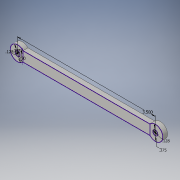
# Autodesk Inventor part: Sun_LinkageArm
Saved by Autodesk Inventor 2016 (Build 200138000, 138)
## iProperties
Created: 2018-01-10
Part Number: Sun_LinkageArm
Material: Generic
Document SubType Name: Modeling
Designer: sun01147
Density: 1 g/cm^3
Appearance: Default
Mass: 2.01542 g
Surface Area: 19.9973 cm^2
Volume: 2.01542 cm^3
Author: sun01147
Autodesk Inventor part; units mm, degrees
ref_plane "YZ Plane" through (0, 0, 0) normal (1, 0, 0) x (0, 1, 0)
ref_plane "XZ Plane" through (0, 0, 0) normal (0, 1, 0) x (-1, 0, 0)
ref_plane "XY Plane" through (0, 0, 0) normal (0, 0, 1) x (1, 0, 0)
sketch "Linkagearm" plane through (0, 0, 0) normal (0, 0, 1) x (1, 0, 0)
  arc A0 (3.5498, 3.175) -> (3.5498, -3.175) centre (0, 0) ccw
  line L0 (3.5498, 3.175) -> (85.3502, 3.175)
  line L1 (85.3502, 3.175) -> (85.3502, -3.175)
  line L2 (85.3502, -3.175) -> (3.5498, -3.175)
  line L3 (3.5498, -3.175) -> (3.5498, 3.175)
  arc A1 (85.3502, -3.175) -> (85.3502, 3.175) centre (88.9, 0) ccw
  circle A2 centre (0, 0) radius 1.6256
  circle A3 centre (88.9, 0) radius 1.6256
  dimension "d0" = 9.525
  dimension "d2" = 6.35
  dimension "d3" = 9.525
  dimension "d4" = 3.2512
  dimension "d5" = 3.2512
  dimension "d8" = 88.9
  constraints: 8 end point, 5 coincident, 4 centre point, 4 point on circle, 2 parallel, 1 horizontal, 1 perpendicular
  measures "d0" diameter of A0
  measures "d2" distance of L2.end L0.start
  measures "d3" diameter of A1
  measures "d4" diameter of A2
  measures "d5" diameter of A3
  measures "d8" distance of A1.centre point (0, 0)
extrude "Extrusion1" add sketch "Linkagearm" against normal blind 3.175
body "Solid1"
